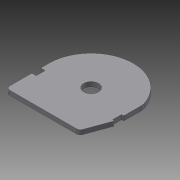
# Autodesk Inventor part: NPT Flange Inner
Saved by Autodesk Inventor 2015 (Build 190159000, 159)
## iProperties
Created: 2015-06-18
Part Number: NPT Flange Inner
Material: Generic
Document SubType Name: Modeling
Designer: JR
Density: 1 g/cm^3
Appearance: Default
Author: JR
Autodesk Inventor part; units mm, degrees
ref_plane "YZ Plane" through (0, 0, 0) normal (1, 0, 0) x (0, 1, 0)
ref_plane "XZ Plane" through (0, 0, 0) normal (0, 1, 0) x (-1, 0, 0)
ref_plane "XY Plane" through (0, 0, 0) normal (0, 0, 1) x (1, 0, 0)
sketch "Sketch1" plane through (0, 0, 0) normal (0, 0, 1) x (1, 0, 0)
  circle A0 centre (0, 0) radius 10
  line L0 (-57, -58) -> (42, -58)
  line L1 (42, -58) -> (54.739, -23)
  line L2 (54.739, -23) -> (52, -23)
  line L3 (52, -23) -> (52, -11)
  line L4 (52, -11) -> (55, -11)
  line L5 (55, -11) -> (55, 12)
  line L6 (-57, -58) -> (-57, -23)
  line L7 (-57, -23) -> (-51, -23)
  line L8 (-51, -23) -> (-51, -11)
  line L9 (-51, -11) -> (-57, -11)
  line L10 (-57, -11) -> (-57, 0)
  arc A1 (53.9189, 18.4865) -> (-57, 0) centre (0, 0) ccw
  arc A2 (55, 12) -> (53.9189, 18.4865) centre (35, 12) ccw
  dimension "d0" = 20
  dimension "d1" = 57
  dimension "d2" = 20
  dimension "d3" = 99
  dimension "d4" = 6
  dimension "d5" = 110
  dimension "d6" = 3
  dimension "d7" = 12
  dimension "d8" = 58
  dimension "d9" = 12
  dimension "d10" = 55
  dimension "d11" = 47
  constraints: 22 end point, 6 perpendicular, 4 point on circle, 3 centre point, 3 tangent, 2 coincident, 2 point on line, 1 collinear, 1 horizontal, 1 parallel, 1 vertical
  measures "d0" diameter of A0
  measures "d1" radius of A1
  measures "d2" radius of A2
  measures "d3" distance of L0.start L0.end
  measures "d4" distance of L6.end L7.end
  measures "d5" angle of L0 L1
  measures "d6" distance of L3.end L4.end
  measures "d7" distance between parallel lines of L2 L4
  measures "d8" distance from line of L0 point (0, 0)
  measures "d9" distance between parallel lines of L7 L9
  measures "d10" distance from line of L5 point (0, 0)
  measures "d11" distance between parallel lines of L0 L9
extrude "Extrusion1" add sketch "Sketch1" along normal blind 6
fillet "Fillet1" radius 0.5 4 edges at (52, -23, 3) (52, -11, 3) (-51, -11, 3) (-51, -23, 3)
fillet "Fillet2" radius 1 4 edges at (-57, -11, 3) (-57, -23, 3) (55, -11, 3) (54.739, -23, 3)
fillet "Fillet3" radius 5 2 edges at (42, -58, 3) (-57, -58, 3)
body "Solid1"
